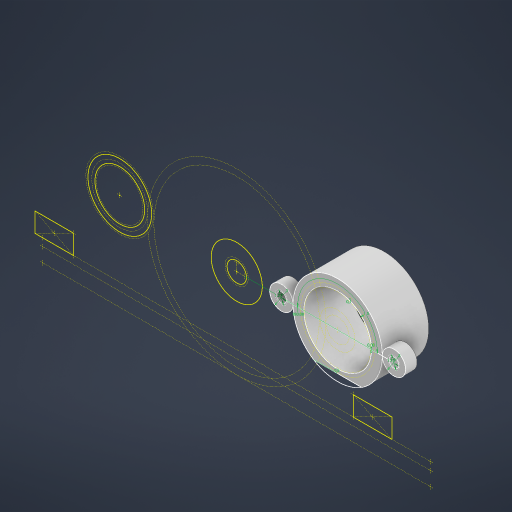
# Autodesk Inventor part: motorsupporter
Saved by Autodesk Inventor 2023.5 (Build 275446000, 446)
## iProperties
Created: 2025-01-19
Part Number: motorsupporter
Material: 一般
Document SubType Name: Modeling
Designer: IshiiLabHonda
Density: 1 g/cm^3
Appearance: 既定
Author: IshiiLabHonda
Autodesk Inventor part; units mm, degrees
ref_plane "YZ Plane" through (0, 0, 0) normal (1, 0, 0) x (0, 1, 0)
ref_plane "XZ Plane" through (0, 0, 0) normal (0, 1, 0) x (-1, 0, 0)
ref_plane "XY Plane" through (0, 0, 0) normal (0, 0, 1) x (1, 0, 0)
derived "motormount-l.ipt"
sketch "スケッチ2" plane through (0, 0, 0) normal (0, 0, 1) x (1, 0, 0)
  circle A0 centre (-15.0669, 1) radius 4.35 construction
  line L0 (0, 0) -> (0, 1) construction
  circle A1 centre (0, 0) radius 10.65 construction
  circle A2 centre (0, 0) radius 11.5 construction
  line L1 (-25, -8.7) -> (25, -8.7) construction
  line L2 (-25, -9.7) -> (25, -9.7) construction
  line L3 (-25, -11.5) -> (25, -11.5) construction
  line L4 (0, 0) -> (1, 0) construction
  circle A3 centre (13, 0) radius 2.25 construction
  circle A4 centre (13, 0) radius 4.25 construction
  circle A5 centre (-15.0669, 1) radius 3.6 construction
  circle A6 centre (-15.0669, 1) radius 3 construction
  circle A7 centre (0, 0) radius 1.25 construction
  circle A8 centre (0, 0) radius 1.5 construction
sketch "スケッチ3" plane through (0, 0, 0) normal (0, 0, 1) x (1, 0, 0)
  circle A0 centre (-15.0669, 1) radius 4.35 construction
  line L0 (0, 0) -> (0, 1) construction
  line L1 (0, 0) -> (1, 0) construction
  line L2 (-25, -11.5) -> (25, -11.5) construction
  line L3 (-25, -9.7) -> (25, -9.7) construction
  line L4 (-25, -8.7) -> (25, -8.7) construction
  circle A1 centre (13, 0) radius 2.25 construction
  circle A2 centre (0, 0) radius 10.65 construction
  circle A3 centre (0, 0) radius 11.5 construction
  circle A4 centre (-15.0669, 1) radius 4.35 construction
  line L5 (0, 0) -> (0, 1) construction
  circle A5 centre (0, 0) radius 10.65 construction
  circle A6 centre (0, 0) radius 11.5 construction
  line L6 (-25, -8.7) -> (25, -8.7) construction
  line L7 (-25, -9.7) -> (25, -9.7) construction
  line L8 (-25, -11.5) -> (25, -11.5) construction
  line L9 (0, 0) -> (1, 0) construction
  circle A7 centre (13, 0) radius 2.25 construction
  circle A8 centre (13, 0) radius 4.25 construction
  circle A9 centre (-15.0669, 1) radius 3.6 construction
  circle A10 centre (-15.0669, 1) radius 3 construction
  line L10 (-26, -6.2) -> (-21, -6.2)
  line L11 (-21, -6.2) -> (-21, -8.7)
  line L12 (-26, -8.7) -> (-26, -6.2)
  line L13 (15, -6.2) -> (20, -6.2)
  line L14 (20, -6.2) -> (20, -8.7)
  line L15 (15, -8.7) -> (15, -6.2)
  line L16 (-26, -6.2) -> (-21, -8.7) construction
  line L17 (-26, -8.7) -> (-21, -6.2) construction
  line L18 (15, -6.2) -> (20, -8.7) construction
  line L19 (15, -8.7) -> (20, -6.2) construction
  line L20 (-26, -8.7) -> (-21, -8.7)
  line L21 (15, -8.7) -> (20, -8.7)
  circle A11 centre (-15.0669, 1) radius 3.2
  circle A12 centre (-15.0669, 1) radius 4.1
  circle A13 centre (13, 0) radius 4.75 construction
  circle A14 centre (0, 0) radius 3.2895
  circle A15 centre (0, 0) radius 1.25
  circle A16 centre (13, 0) radius 1.5 construction
  point P0 (-23.5, -7.45)
  point P1 (17.5, -7.45)
sketch "スケッチ5" plane through (0, 0, 0) normal (0, 0, 1) x (1, 0, 0)
  circle A0 centre (-15.0669, 1) radius 4.35 construction
  line L0 (0, 0) -> (0, 1) construction
  circle A1 centre (0, 0) radius 10.65 construction
  circle A2 centre (0, 0) radius 11.5 construction
  line L1 (-25, -8.7) -> (25, -8.7) construction
  line L2 (-25, -9.7) -> (25, -9.7) construction
  line L3 (-25, -11.5) -> (25, -11.5) construction
  line L4 (0, 0) -> (1, 0) construction
  circle A3 centre (13, 0) radius 2.25 construction
  circle A4 centre (13, 0) radius 4.25 construction
  circle A5 centre (-15.0669, 1) radius 3.6 construction
  circle A6 centre (-15.0669, 1) radius 3 construction
  circle A7 centre (0, 0) radius 1.25 construction
  circle A8 centre (0, 0) radius 1.5 construction
  circle A9 centre (0, 0) radius 10.65 construction
  line L5 (0, 0) -> (0, 1) construction
  line L6 (0, 0) -> (1, 0) construction
  circle A10 centre (13, 0) radius 2.25 construction
  circle A11 centre (-15.0669, 1) radius 4.35 construction
  circle A12 centre (0, 0) radius 11.5 construction
  line L7 (-25, -11.5) -> (25, -11.5) construction
  line L8 (-25, -9.7) -> (25, -9.7) construction
  line L9 (-25, -8.7) -> (25, -8.7) construction
  circle A13 centre (13, 0) radius 2.25 construction
  circle A14 centre (13, 0) radius 1.5 construction
  circle A15 centre (13, 0) radius 2.25 construction
  circle A16 centre (13, 0) radius 4.75 construction
  line L10 (15, -8.7) -> (15, -6.2) projected
  line L11 (20, -6.2) -> (20, -8.7) projected
  line L12 (15, -6.2) -> (20, -8.7) construction
  line L13 (15, -8.7) -> (20, -8.7) projected
  line L14 (15, -8.7) -> (20, -6.2) construction
  line L15 (15, -6.2) -> (20, -6.2) projected
  circle A17 centre (13, 0) radius 4.25 construction
  circle A18 centre (-15.0669, 1) radius 4.35 construction
  line L16 (0, 0) -> (0, 1) construction
  line L17 (0, 0) -> (1, 0) construction
  line L18 (-25, -11.5) -> (25, -11.5) construction
  line L19 (-25, -9.7) -> (25, -9.7) construction
  line L20 (-25, -8.7) -> (25, -8.7) construction
  line L21 (0, 0) -> (0, 1) construction
  line L22 (0, 0) -> (1, 0) construction
  line L23 (-25, -8.7) -> (25, -8.7) construction
  line L24 (-25, -9.7) -> (25, -9.7) construction
  line L25 (-25, -11.5) -> (25, -11.5) construction
  circle A19 centre (0, 0) radius 11.5 construction
  circle A20 centre (0, 0) radius 11.5 construction
  circle A21 centre (0, 0) radius 10.65 construction
  circle A22 centre (0, 0) radius 10.65 construction
  circle A23 centre (0, 0) radius 1.25 projected
  circle A24 centre (0, 0) radius 3.2895 projected
  circle A25 centre (-15.0669, 1) radius 4.35 construction
  circle A26 centre (-15.0669, 1) radius 3.6 construction
  circle A27 centre (-15.0669, 1) radius 3 construction
  circle A28 centre (-15.0669, 1) radius 3.2 projected
  circle A29 centre (-15.0669, 1) radius 4.1 projected
  line L26 (-21, -6.2) -> (-21, -8.7) projected
  line L27 (-26, -6.2) -> (-21, -6.2) projected
  line L28 (-26, -6.2) -> (-21, -8.7) construction
  line L29 (-26, -8.7) -> (-21, -6.2) construction
  line L30 (-26, -8.7) -> (-21, -8.7) projected
  line L31 (-26, -8.7) -> (-26, -6.2) projected
  circle A30 centre (13, 0) radius 5.75
  circle A31 centre (20.25, 0) radius 0.625
  circle A32 centre (20.25, 0) radius 1.5
  circle A33 centre (20.25, 0) radius 0.8 construction
  circle A34 centre (5.75, 0) radius 0.625
  circle A35 centre (5.75, 0) radius 1.5
  circle A36 centre (5.75, 0) radius 0.8 construction
  circle A37 centre (13, 0) radius 4.35
  line L32 (13, 0) -> (20.25, 0)
  line L33 (13, 0) -> (5.75, 0)
  line L34 (9.9113, -4.85) -> (16.0887, -4.85)
  point P0 (17.5, -7.45)
  point P1 (-23.5, -7.45)
  dimension "d1" = 1.5
  dimension "d2" = 1.25
  dimension "d3" = 3
  dimension "d4" = 1.6
  dimension "d5" = 1.25
  dimension "d6" = 3
  dimension "d7" = 1.6
  dimension "d10" = 0.1
  dimension "d13" = 0
  dimension "d14" = 0
  dimension "d15" = 0.5
  constraints: 8 centre point, 6 coincident, 6 end point, 2 point on circle, 2 tangent, 1 parallel, 11 other
  measures "d1" radial gap between concentric circles of A30 A4
  measures "d2" diameter of A31
  measures "d3" diameter of A32
  measures "d4" diameter of A33
  measures "d5" diameter of A34
  measures "d6" diameter of A35
  measures "d7" diameter of A36
  measures "d10" radial gap between concentric circles of A4 A37
  measures "d13" vertical extent of L32
  measures "d14" vertical extent of L33
  measures "d15" distance edge to line of A37 L34
extrude "押し出し1" add sketch "スケッチ5" against normal blind 1.5 contours A35 | A32
extrude "押し出し2" add sketch "スケッチ5" against normal blind 6 contours L32 A37 L33 A30 | A30 L34 L33 A37 L32 | A30 L34
extrude "押し出し3" cut sketch "スケッチ5" against normal blind 10 contours A30 L34
sketch "スケッチ1" plane through (0, 0, 0) normal (0, 0, 1) x (1, 0, 0)
  circle A0 centre (0, 0) radius 10.65 construction
  line L0 (0, 0) -> (0, 1) construction
  line L1 (0, 0) -> (1, 0) construction
  circle A1 centre (13, 0) radius 2.25 construction
  circle A2 centre (-15.0669, 1) radius 4.35 construction
  circle A3 centre (0, 0) radius 11.5 construction
  line L2 (-25, -11.5) -> (25, -11.5) construction
  line L3 (-25, -9.7) -> (25, -9.7) construction
  line L4 (-25, -8.7) -> (25, -8.7) construction
